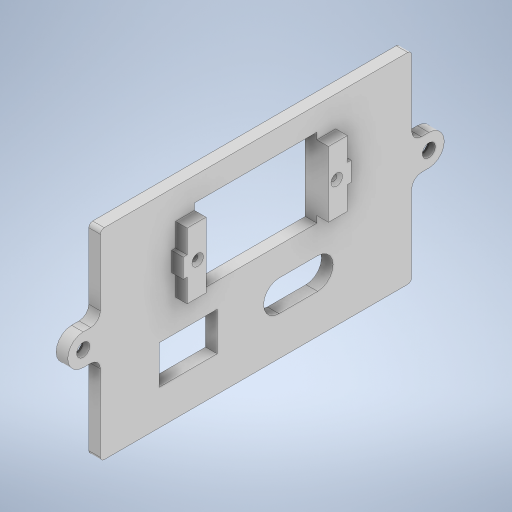
# Autodesk Inventor part: pokrywa_tyl
Saved by Autodesk Inventor 2023.4 (Build 274418000, 418)
## iProperties
Created: 2024-07-28
Part Number: pokrywa_tyl
Material: Ogólny
Document SubType Name: Modeling
Designer: kamil
Density: 1 g/cm^3
Appearance: Domyślna
Author: kamil
Autodesk Inventor part; units mm, degrees
ref_plane "YZ Plane" through (0, 0, 0) normal (1, 0, 0) x (0, 1, 0)
ref_plane "XZ Plane" through (0, 0, 0) normal (0, 1, 0) x (-1, 0, 0)
ref_plane "XY Plane" through (0, 0, 0) normal (0, 0, 1) x (1, 0, 0)
sketch "Szkic1" plane through (0, 0, 0) normal (1, 0, 0) x (0, 1, 0)
  line L0 (-29.4319, -23.6453) -> (19.8681, -23.6453)
  line L1 (19.8681, -23.6453) -> (19.8681, 56.9547)
  line L2 (19.8681, 56.9547) -> (-29.4319, 56.9547)
  line L3 (-29.4319, 56.9547) -> (-29.4319, -23.6453)
  point P0 (0, 0)
  dimension "d0" = 80.6
  dimension "d1" = 49.3
  constraints: 8 end point, 2 parallel, 1 horizontal, 1 perpendicular
  measures "d0" distance of L0.end L1.end
  measures "d1" distance between parallel lines of L3 L1
extrude "Wyciągnięcie proste1" add sketch "Szkic1" along normal blind 3
sketch "Sketch6" plane through (0, 0, 0) normal (-1, 0, 0) x (0, 0, 1)
  arc A0 (-28.0945, -0.5319) -> (-28.0945, -9.0319) centre (-28.0945, -4.7819) ccw
  line L0 (-26.3445, -9.0319) -> (-28.0945, -9.0319)
  line L1 (-26.3445, -0.5319) -> (-28.0945, -0.5319)
  line L2 (59.654, -6.3319) -> (61.404, -6.3319)
  arc A1 (61.404, -6.3319) -> (61.404, 2.1681) centre (61.404, -2.0819) ccw
  line L3 (59.654, 2.1681) -> (61.404, 2.1681)
  line L4 (-23.6453, 19.8681) -> (56.9547, 19.8681)
  line L5 (-23.6453, -29.4319) -> (-23.6453, 19.8681)
  line L6 (56.9547, -29.4319) -> (-23.6453, -29.4319)
  line L7 (56.9547, 19.8681) -> (56.9547, -29.4319)
  line L8 (-26.3445, -8.7819) -> (-28.0945, -8.7819)
  arc A2 (-28.0945, -0.7819) -> (-28.0945, -8.7819) centre (-28.0945, -4.7819) ccw
  line L9 (-28.0945, -0.7819) -> (-26.3445, -0.7819)
  line L10 (-26.3445, -0.7819) -> (-23.6453, -0.7819)
  line L11 (-23.6453, -29.4319) -> (-23.6453, 19.8681)
  line L12 (-26.3445, -8.7819) -> (-23.6453, -8.7819)
  line L13 (-23.6453, 19.8681) -> (56.9547, 19.8681)
  line L14 (16.6547, 19.8681) -> (16.6547, -29.4319)
  line L15 (56.9547, -29.4319) -> (-23.6453, -29.4319)
  line L16 (59.654, -8.7819) -> (61.404, -8.7819)
  arc A3 (61.404, -8.7819) -> (61.404, -0.7819) centre (61.404, -4.7819) ccw
  line L17 (61.404, -0.7819) -> (59.654, -0.7819)
  line L18 (59.654, -0.7819) -> (56.9547, -0.7819)
  line L19 (59.654, -8.7819) -> (56.9547, -8.7819)
  point P0 (0, 0)
extrude "Extrusion4" add sketch "Sketch6" against normal blind 3 contours L5 L12 L8 A2 L9 L10 | L18 L17 A3 L16 L19 L7
fillet "Fillet2" radius 2.5 4 edges at (1.5, -0.7819, -23.6453) (1.5, -8.7819, -23.6453) (1.5, -0.7819, 56.9547) (1.5, -8.7819, 56.9547)
sketch "Sketch8" plane through (0, 0, 0) normal (-1, 0, 0) x (0, 0, 1)
  line L0 (32.3929, 13.5523) -> (1.0929, 13.5523) projected
  line L1 (1.0929, 13.5523) -> (1.0929, -6.4477) projected
  line L2 (1.0929, -6.4477) -> (32.3929, -6.4477) projected
  line L3 (32.3929, -6.4477) -> (32.3929, 13.5523) projected
  line L4 (0.8929, -6.6477) -> (0.8929, 13.7523)
  line L5 (0.8929, 13.7523) -> (32.5929, 13.7523)
  line L6 (32.5929, 13.7523) -> (32.5929, -6.6477)
  line L7 (32.5929, -6.6477) -> (0.8929, -6.6477)
  point P0 (0, 0)
  dimension "d38" = 0.2
  constraints: 8 end point, 3 other
  measures "d38" distance between parallel lines of L1 L4
extrude "Extrusion5" cut sketch "Sketch8" against normal blind 3 contours L3 L2 L1 L0 | L4 L5 L6 L7
sketch "Sketch9" plane through (3, 0, 0) normal (1, 0, 0) x (0, 0, -1)
  line L0 (-32.5929, 13.7523) -> (-0.8929, 13.7523) projected
  line L1 (-0.8929, 13.7523) -> (-0.8929, -6.6477) projected
  line L2 (-0.8929, -6.6477) -> (-32.5929, -6.6477) projected
  line L3 (-32.5929, -6.6477) -> (-32.5929, 13.7523) projected
  line L4 (-56.9547, -29.4319) -> (23.6453, -29.4319) projected
  line L5 (23.6453, -29.4319) -> (23.6453, -11.2819) projected
  arc A0 (26.1453, -8.7819) -> (23.6453, -11.2819) centre (26.1453, -11.2819) ccw projected
  line L6 (26.1453, -8.7819) -> (28.0945, -8.7819) projected
  arc A1 (28.0945, -8.7819) -> (28.0945, -0.7819) centre (28.0945, -4.7819) ccw projected
  line L7 (28.0945, -0.7819) -> (26.1453, -0.7819) projected
  arc A2 (23.6453, 1.7181) -> (26.1453, -0.7819) centre (26.1453, 1.7181) ccw projected
  line L8 (23.6453, 1.7181) -> (23.6453, 19.8681) projected
  line L9 (23.6453, 19.8681) -> (-56.9547, 19.8681) projected
  line L10 (-56.9547, 19.8681) -> (-56.9547, 1.7181) projected
  line L11 (-37.4929, 12.0523) -> (-37.4929, 6.0523) projected
  line L12 (-37.4929, 6.0523) -> (-38.4929, 6.0523) projected
  line L13 (-38.4929, 6.0523) -> (-38.4929, 1.0523) projected
  line L14 (-38.4929, 1.0523) -> (-37.4929, 1.0523) projected
  line L15 (-37.4929, 1.0523) -> (-37.4929, -4.9477) projected
  line L16 (-37.4929, -4.9477) -> (4.0071, -4.9477) projected
  line L17 (4.0071, -4.9477) -> (4.0071, 1.0523) projected
  line L18 (4.0071, 1.0523) -> (5.0071, 1.0523) projected
  line L19 (5.0071, 1.0523) -> (5.0071, 6.0523) projected
  line L20 (5.0071, 6.0523) -> (4.0071, 6.0523) projected
  line L21 (4.0071, 6.0523) -> (4.0071, 12.0523) projected
  line L22 (4.0071, 12.0523) -> (-37.4929, 12.0523) projected
  circle A3 centre (1.2571, 3.5523) radius 1.2 projected
  circle A4 centre (-34.7429, 3.5523) radius 1.2 projected
  line L23 (-59.4547, -0.7819) -> (-61.404, -0.7819) projected
  arc A5 (-61.404, -0.7819) -> (-61.404, -8.7819) centre (-61.404, -4.7819) ccw projected
  line L24 (-61.404, -8.7819) -> (-59.4547, -8.7819) projected
  line L25 (-56.9547, -11.2819) -> (-56.9547, -29.4319) projected
  arc A6 (-59.4547, -0.7819) -> (-56.9547, 1.7181) centre (-59.4547, 1.7181) ccw projected
  arc A7 (-56.9547, -11.2819) -> (-59.4547, -8.7819) centre (-59.4547, -11.2819) ccw projected
  point P0 (0, 0)
  point P1 (-0.8929, 12.0523)
  point P2 (-0.8929, -4.9477)
  point P3 (-32.5929, -4.9477)
  point P4 (-32.5929, 12.0523)
ref_plane "Work Plane2" through (6, -4.9477, 32.3929) normal (-1, 0, 0) x (0, 0, 1)
extrude "Extrusion6" add sketch "Sketch9" along normal up to surface (3 mm away) contours L3 L16 L15 L14 L13 L12 L11 L22 | L22 L21 L20 L19 L18 L17 L16 L1 | A3 | A4
sketch "Sketch10" plane through (6, -4.9477, 32.5929) normal (1, 0, 0) x (0, 0, -1)
  circle A0 centre (33.85, 8.5) radius 1.2 projected
  circle A1 centre (-2.15, 8.5) radius 1.2 projected
  point P0 (32.5929, 4.9477)
hole "Hole4" at (6, 3.5523, -1.2571) at (6, 3.5523, 34.7429) direction (-1, 0, 0) diameter 1.5 depth 5 tip angle 118 countersink diameter 3 countersink angle 90
sketch "Sketch11" plane through (3, 0, 0) normal (1, 0, 0) x (0, 0, -1)
  line L0 (-56.9547, -29.4319) -> (23.6453, -29.4319) projected
  line L1 (23.6453, -29.4319) -> (23.6453, -11.2819) projected
  arc A0 (26.1453, -8.7819) -> (23.6453, -11.2819) centre (26.1453, -11.2819) ccw projected
  line L2 (26.1453, -8.7819) -> (28.0945, -8.7819) projected
  arc A1 (28.0945, -8.7819) -> (28.0945, -0.7819) centre (28.0945, -4.7819) ccw projected
  line L3 (28.0945, -0.7819) -> (26.1453, -0.7819) projected
  arc A2 (23.6453, 1.7181) -> (26.1453, -0.7819) centre (26.1453, 1.7181) ccw projected
  line L4 (23.6453, 1.7181) -> (23.6453, 19.8681) projected
  line L5 (23.6453, 19.8681) -> (-56.9547, 19.8681) projected
  line L6 (-56.9547, 19.8681) -> (-56.9547, 1.7181) projected
  line L7 (-0.8929, 12.0523) -> (4.0071, 12.0523) projected
  line L8 (4.0071, 12.0523) -> (4.0071, 6.0523) projected
  line L9 (4.0071, 6.0523) -> (5.0071, 6.0523) projected
  line L10 (5.0071, 6.0523) -> (5.0071, 1.0523) projected
  line L11 (5.0071, 1.0523) -> (4.0071, 1.0523) projected
  line L12 (4.0071, 1.0523) -> (4.0071, -4.9477) projected
  line L13 (4.0071, -4.9477) -> (-0.8929, -4.9477) projected
  line L14 (-0.8929, -4.9477) -> (-0.8929, -6.6477) projected
  line L15 (-0.8929, -6.6477) -> (-32.5929, -6.6477) projected
  line L16 (-32.5929, -6.6477) -> (-32.5929, -4.9477) projected
  line L17 (-32.5929, -4.9477) -> (-37.4929, -4.9477) projected
  line L18 (-37.4929, -4.9477) -> (-37.4929, 1.0523) projected
  line L19 (-37.4929, 1.0523) -> (-38.4929, 1.0523) projected
  line L20 (-38.4929, 1.0523) -> (-38.4929, 6.0523) projected
  line L21 (-38.4929, 6.0523) -> (-37.4929, 6.0523) projected
  line L22 (-37.4929, 6.0523) -> (-37.4929, 12.0523) projected
  line L23 (-37.4929, 12.0523) -> (-32.5929, 12.0523) projected
  line L24 (-32.5929, 12.0523) -> (-32.5929, 13.7523) projected
  line L25 (-32.5929, 13.7523) -> (-0.8929, 13.7523) projected
  line L26 (-0.8929, 13.7523) -> (-0.8929, 12.0523) projected
  line L27 (-41.6988, -13.0398) -> (-26.6988, -13.0398)
  line L28 (-26.6988, -13.0398) -> (-26.6988, -23.0398)
  line L29 (-26.6988, -23.0398) -> (-41.6988, -23.0398)
  line L30 (-41.6988, -23.0398) -> (-41.6988, -13.0398)
  line L31 (-10.6988, -18.0398) -> (-0.6988, -18.0398) construction
  line L32 (-10.6988, -22.0398) -> (-0.6988, -22.0398)
  line L33 (-0.6988, -14.0398) -> (-10.6988, -14.0398)
  arc A3 (-10.6988, -14.0398) -> (-10.6988, -22.0398) centre (-10.6988, -18.0398) ccw
  arc A4 (-0.6988, -22.0398) -> (-0.6988, -14.0398) centre (-0.6988, -18.0398) ccw
  line L34 (-26.6988, -18.0398) -> (-6.6988, -18.0398) construction
  line L35 (-0.8929, -6.6477) -> (-32.5929, -6.6477) construction
  line L36 (-16.7429, -6.6477) -> (-16.6547, -29.4319) construction
  line L37 (-55.9547, -29.4319) -> (22.6453, -29.4319) construction
  line L38 (-59.4547, -0.7819) -> (-61.404, -0.7819) projected
  arc A5 (-61.404, -0.7819) -> (-61.404, -8.7819) centre (-61.404, -4.7819) ccw projected
  line L39 (-61.404, -8.7819) -> (-59.4547, -8.7819) projected
  line L40 (-56.9547, -11.2819) -> (-56.9547, -29.4319) projected
  arc A6 (-59.4547, -0.7819) -> (-56.9547, 1.7181) centre (-59.4547, 1.7181) ccw projected
  arc A7 (-56.9547, -11.2819) -> (-59.4547, -8.7819) centre (-59.4547, -11.2819) ccw projected
  point P0 (0, 0)
  point P1 (-5.6988, -18.0398)
  point P2 (-16.6988, -18.0398)
  dimension "d50" = 10
  dimension "d51" = 15
  dimension "d53" = 20
  dimension "d54" = 10
  dimension "d55" = 8
  constraints: 20 end point, 6 midpoint, 5 point on circle, 4 parallel, 4 tangent, 2 centre point, 2 horizontal, 1 perpendicular
  measures "d50" distance between parallel lines of L29 L27
  measures "d51" distance between parallel lines of L28 L30
  measures "d53" distance of L34.start L34.end
  measures "d54" distance of L31.start L31.end
  measures "d55" distance between parallel lines of L32 L33
extrude "Extrusion7" cut sketch "Sketch11" against normal through all contours L27 L28 L29 L30 | A3 L33 A4 L32
sketch "Sketch12" plane through (0, 0, 0) normal (-1, 0, 0) x (0, 0, 1)
  arc A0 (-28.0945, -0.7819) -> (-28.0945, -8.7819) centre (-28.0945, -4.7819) ccw projected
  arc A1 (61.404, -8.7819) -> (61.404, -0.7819) centre (61.404, -4.7819) ccw projected
  point P0 (0, 0)
hole "Hole5" at (0, -4.7819, -28.0945) at (0, -4.7819, 61.404) direction (1, 0, 0) diameter 3.4 depth 10 countersink diameter 6 countersink angle 90
sketch "Sketch13" plane through (0, -29.4319, -23.6453) normal (0, -1, 0) x (1, 0, 0)
  line L0 (0, 80.6) -> (0, 0) projected
  line L1 (0, 0) -> (3, 0) projected
  line L2 (3, 80.6) -> (3, 0) projected
  line L3 (0, 80.6) -> (3, 80.6) projected
  point P0 (0, 23.6453)
extrude "Extrusion8" add sketch "Sketch13" along normal blind 2.7
fillet "Fillet4" radius 1 4 edges at (1.5, -32.1319, -23.6453) (1.5, -32.1319, 56.9547) (1.5, 19.8681, -23.6453) (1.5, 19.8681, 56.9547)
